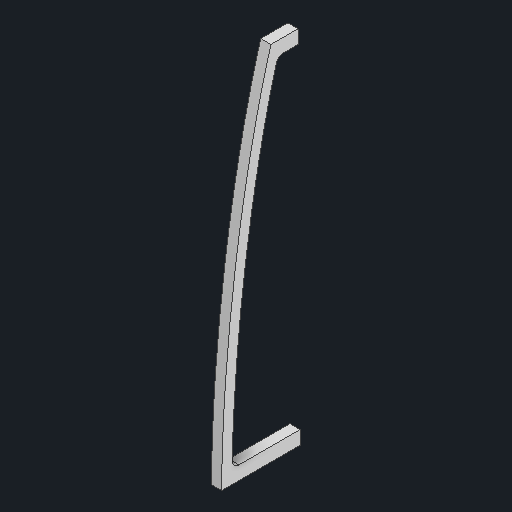
# Autodesk Inventor part: nose_spanner
Saved by Autodesk Inventor 2024 (Build 280153000, 153)
## iProperties
Created: 2022-07-02
Part Number: nose_spanner
Material: Generic
Document SubType Name: Modeling
Designer: kardo
Density: 1 g/cm^3
Appearance: Default
Mass: 1.2776 g
Surface Area: 16.635 cm^2
Volume: 1.2776 cm^3
Author: kardo
Autodesk Inventor part; units mm, degrees
ref_plane "YZ Plane" through (0, 0, 0) normal (1, 0, 0) x (0, 1, 0)
ref_plane "XZ Plane" through (0, 0, 0) normal (0, 1, 0) x (-1, 0, 0)
ref_plane "XY Plane" through (0, 0, 0) normal (0, 0, 1) x (1, 0, 0)
derived "surface_body.ipt"
sketch "sk_rail_top_tunnel" plane through (81.12, 0, 0) normal (1, 0, 0) x (0, 1, 0)
  line L0 (255, 107.6209) -> (255, -224.5198)
  line L1 (0, 107.6209) -> (0, -224.5198)
  line L2 (-345, 107.6209) -> (-345, -224.5198)
  line L3 (-345, 0) -> (0, 0)
  line L4 (-172.5, 48.8998) -> (-172.5, 0)
  line L5 (0, 52.89) -> (37.026, 52.89)
  line L6 (37.026, 52.89) -> (80.784, 47.0555)
  line L7 (80.784, 47.0555) -> (112.2, 37.536)
  line L8 (112.2, 107.6209) -> (112.2, -224.5198)
  line L9 (0, 52.89) -> (255, 52.89)
  line L10 (-469.9275, 0) -> (379.2584, 0)
  spline S0 degree 3 poles (0, 52.89) (92.8353, 52.89) (195.0311, 49.5089) (255, 36.448) knots 0 0 0 0 1 1 1 1
  spline S1 degree 3 poles (0, 52.89) (37.026, 52.89) (80.784, 47.0555) (112.2, 37.536) knots 1 1 1 1 2 2 2 2
  spline S2 degree 4 poles (-345, 37.3935) (-258.8686, 45.1235) (-172.5923, 49.7074) (-86.3167, 52.89) (0, 52.89) knots 0 0 0 0 0 1 1 1 1 1
  point P0 (153, 48.7795)
  point P1 (112.2, 28.832)
  point P2 (-230.0001, 45.8224)
  point P3 (-114.9999, 50.9907)
sketch "sk_rail_bottom_tunnel" plane through (81.12, 0, 0) normal (1, 0, 0) x (0, 1, 0)
  line L0 (-241.5001, 19.2432) -> (11.22, 28.376)
  arc A0 (36.465, 28.832) -> (11.22, 28.376) centre (36.465, -670.197) ccw
  line L1 (36.465, 28.832) -> (112.2, 28.832)
  arc A1 (-262.2001, 18.586) -> (-241.5001, 19.2432) centre (-326.8578, 2381.2399) ccw
  line L2 (-345, 16.32) -> (-262.2001, 18.586)
  point P0 (0, 0)
ref_plane "plane_tunnel_right" through (81.12, 0, 0) normal (1, 0, 0) x (0, 1, 0)
ref_plane "plane_middle" through (0, 0, 0) normal (0, 1, 0) x (-1, 0, 0)
derived "parameters_frame.ipt"
sketch "sk_base" plane through (81.12, 0, 0) normal (1, 0, 0) x (0, 1, 0)
  spline S0 degree 3 poles (0, 52.89) (37.026, 52.89) (80.784, 47.0555) (112.2, 37.536) knots 1 1 1 1 2 2 2 2 construction
  line L0 (36.465, 28.832) -> (112.2, 28.832) construction
  arc A0 (36.465, 28.832) -> (11.22, 28.376) centre (36.465, -670.197) ccw construction
  line L1 (-241.5001, 19.2432) -> (11.22, 28.376) construction
  line L2 (0, 2991.5273) -> (0, -1280.4843) construction
  line L3 (109.2, 37.5904) -> (109.2, 29.632)
  line L4 (109.2, 29.632) -> (105.2, 29.632)
  line L5 (105.2, 35.6027) -> (105.2, 29.632)
  line L6 (109.2, 29.632) -> (109.2, 28.832) construction
  line L7 (112.2, 37.536) -> (112.2, 28.832) construction
  line L8 (3, 52.0774) -> (3, 28.8795)
  line L9 (3, 28.8795) -> (7, 29.024)
  line L10 (7, 29.024) -> (7, 49.0218)
  line L11 (7, 29.024) -> (7.0289, 28.2245)
  line L12 (3, 28.8795) -> (3.0289, 28.08)
  spline S1 degree 5 poles (3, 52.0773) (14.0563, 51.9848) (25.1086, 51.4746) (36.1391, 50.6354) (57.5264, 48.386) (78.745, 44.8841) (88.9918, 42.8634) (99.1727, 40.4944) (109.2, 37.5902) knots 0 0 0 0 0 0 0.51436 0.51436 0.51436 1 1 1 1 1 1
  spline S2 degree 5 poles (7, 49.0218) (17.1736, 48.8263) (27.3406, 48.2899) (37.488, 47.4744) (57.2505, 45.3513) (76.868, 42.1513) (86.3894, 40.3134) (95.8548, 38.1766) (105.2, 35.6026) knots 0 0 0 0 0 0 0.512135 0.512135 0.512135 1 1 1 1 1 1
  point P0 (0, 0)
  dimension "d3" = 3.8
  dimension "d11" = 0.8
  dimension "d5" = 4
  dimension "d6" = 0.8
  dimension "d7" = 3
  dimension "d8" = 3
  dimension "d9" = 4
  dimension "d10" = 0.8
  constraints: 20 end point, 6 parallel, 3 perpendicular, 3 point on line, 6 other
  measures "d5" distance between parallel lines of L3 L5
  measures "d6" distance of L3.end L6.end
  measures "d7" distance between parallel lines of L7 L3
  measures "d8" distance between parallel lines of L2 L8
  measures "d9" distance between parallel lines of L8 L10
  measures "d10" distance of L9.end L11.end
extrude "Extrusion1" add sketch "sk_base" against normal blind 3
fillet "Fillet1" radius 2 2 edges at (79.62, 105.2, 35.6026) (79.62, 7, 49.0218)
equation "\"d3\" = shell_thickness + 0.75 * bulkhead_inset"
equation "\"d11\" = shell_thickness"
equation "\"d5\" = bulkhead_inset"
equation "\"d6\" = shell_thickness"
equation "\"d7\" = bulkhead_thickness"
equation "\"d8\" = bulkhead_thickness"
equation "\"d9\" = bulkhead_inset"
equation "\"d10\" = shell_thickness"
equation "\"d12\" = bulkhead_thickness"
equation "\"d14\" = 0.5 * bulkhead_inset"
equation "\"shell_thickness\" = 0.8"
equation "\"bulkhead_inset\" = 4"
equation "\"bulkhead_thickness\" = 3"
body "Solid1"
